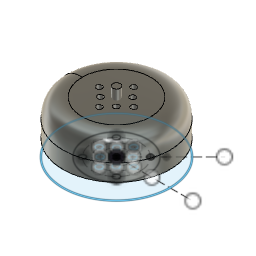
T-MotorMN5008 v1 (Autodesk Fusion 360 design; units mm, degrees)
Autodesk Fusion 360 part; units mm, degrees
sketch "TopSketch" plane through (0, 0, 0) normal (0, 0, 1) x (1, 0, 0) in component "Stator"
  circle A0 centre (0, 0) radius 12.5 construction
  line L0 (0, 0) -> (28.0713, 28.0713) construction
  line L1 (0, 0) -> (39.6989, 0) construction
  circle A1 centre (8.8388, 8.8388) radius 1.5
  circle A2 centre (-8.8388, 8.8388) radius 1.5
  circle A3 centre (-8.8388, -8.8388) radius 1.5
  circle A4 centre (8.8388, -8.8388) radius 1.5
  circle A5 centre (0, 0) radius 16
  circle A6 centre (0, 0) radius 27.8
  dimension "d1" = 25
  dimension "d2" = 45
  dimension "d3" = 3
  dimension "d5" = 360
  dimension "d7" = 32
  dimension "d15" = 55.6
  constraint coincident A0.centre L0.start
  constraint horizontal L1
  constraint coincident A0 A1.centre
  constraint coincident L0 A1.centre
  constraint concentric A5 A6
  measures "d1" diameter of A0
  measures "d2" angle of L0 L1
  measures "d3" diameter of A1
  measures "d7" diameter of A5
  measures "d15" diameter of A6
sketch "FrontSketch" plane through (0, 0, 0) normal (0, 1, 0) x (1, 0, 0) in component "Stator"
  line L0 (-27.8, -27) -> (-27.8, -8.25)
  line L1 (27.8, -27) -> (27.8, -8.25)
  line L2 (0, -23) -> (0, 11) construction
  line L3 (-27.8, -27) -> (27.8, -27)
  line L4 (-27.8, -8.25) -> (27.8, -8.25)
  line L5 (-16, 0) -> (16, 0)
  line L6 (7, -32) -> (-10, -32)
  line L7 (-16, 0) -> (-16, -8.25)
  line L8 (16, 0) -> (16, -8.25)
  dimension "d8" = 27.8
  dimension "d9" = 27.8
  dimension "d10" = 8.25
  dimension "d11" = 27
  dimension "d12" = 32
  constraint vertical L0
  constraint vertical L1
  constraint vertical L2
  constraint coincident origin L2
  constraint horizontal L3
  constraint perpendicular L0 L4
  constraint horizontal L6
  constraint coincident L5.start L7.start
  constraint coincident L4 L7.end
  constraint perpendicular L4 L7
  constraint coincident L5.end L8.start
  constraint coincident L4 L8.end
  constraint perpendicular L4 L8
  measures "d8" distance of L0 L2
  measures "d9" distance of L1 L2
  measures "d10" distance of L4 L5
  measures "d11" distance of L3 L5
  measures "d12" distance of L5 L6
sketch "TopSketch (2)" plane through (0, 0, 0) normal (0, 0, 1) x (1, 0, 0) in component "Rotor"
  circle A0 centre (0, 0) radius 27.8
  circle A1 centre (0, 0) radius 2
  circle A2 centre (0, 0) radius 9 construction
  circle A3 centre (0, 0) radius 6 construction
  circle A4 centre (0, 9) radius 1.5
  line L0 (0, 0) -> (13, 13) construction
  line L1 (0, 0) -> (18.3848, 0) construction
  circle A5 centre (-4.2996, -4.1849) radius 1.5
  circle A6 centre (-9, 0) radius 1.5
  circle A7 centre (4.1849, -4.2996) radius 1.5
  circle A8 centre (0, -9) radius 1.5
  circle A9 centre (4.2996, 4.1849) radius 1.5
  circle A10 centre (9, 0) radius 1.5
  circle A11 centre (-4.1849, 4.2996) radius 1.5
  dimension "d16" = 4
  dimension "d17" = 18
  dimension "d18" = 12
  dimension "d19" = 3
  dimension "d21" = 45
  dimension "d22" = 18.3848
  dimension "d23" = 3
  dimension "d25" = 360
  constraint coincident A0.centre A1.centre
  constraint concentric A0 A1
  constraint concentric A1 A2
  constraint concentric A1 A3
  constraint coincident A2 A4.centre
  constraint horizontal L1
  constraint coincident A3 A5.centre
  measures "d16" diameter of A1
  measures "d17" diameter of A2
  measures "d18" diameter of A3
  measures "d19" diameter of A4
  measures "d21" angle of L0 L1
  measures "d22" distance of A0.centre L0.end
  measures "d23" diameter of A5
extrude "Extrude1" add sketch "TopSketch (2)" along normal blind 27 and the other way blind -8.25 contours A0 | A1 makes body 1 in component "Rotor"
extrude "Extrude2" add sketch "TopSketch (2)" along normal blind 32 and the other way blind -9 separate body contours A1 makes body 2 in component "Rotor"
extrude "Extrude2'" add sketch "TopSketch" along normal blind 9 separate body contours A5 makes body 3 in component "Stator"
fillet "Fillet1" radius 10 tangency weight 1.63045 1 edges at (-25.9187, -10.0529, 27) on bodies 1 in component "Rotor"
extrude "Extrude1'" [suppressed] in component "Stator"
component "Stator" placed x (1, 0, 0) y (0, 1, 0) z (0, 0, 1) at (0, 0, 0)
component "Rotor" placed x (1, 0, 0) y (0, 1, 0) z (0, 0, 1) at (0, 0, 0)
equation "d8 = ( 55.6 / 2 ) * 1 mm"
